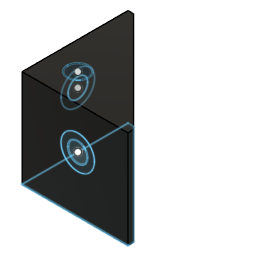
Electronics panel corner connector (Autodesk Fusion 360 design; units mm, degrees)
Autodesk Fusion 360 part; units mm, degrees
note: some values were not read from the file. Chosen so that the rebuilt part matches the saved one: which pieces of a blend or face edit are solid.
sketch "sketch 863" plane through (0, 28.398, 0) normal (0, -1, 0) x (-1, 0, 0)
  line L0 (-91, -772.5) -> (-73, -754.5)
  line L1 (-91, -773.5) -> (-91, -772.5)
  line L2 (-72, -773.5) -> (-91, -773.5)
  line L3 (-72, -773.5) -> (-91, -773.5)
  line L4 (-72, -754.5) -> (-72, -773.5)
  line L5 (-72, -754.5) -> (-72, -773.5)
  line L6 (-73, -754.5) -> (-72, -754.5)
extrude "Extrude1" add sketch "sketch 863" against normal blind 17.5
sketch "sketch 846" plane through (0, 45.898, 0) normal (0, 1, 0) x (-1, 0, 0)
  circle A0 centre (-77, 768.5) radius 1.875
extrude "Extrude2" cut sketch "sketch 846" against normal blind 7.5
sketch "sketch 893" plane through (0, 0, 773.5) normal (0, 0, 1) x (1, 0, 0)
  circle A0 centre (82, 38.398) radius 1.75
extrude "Extrude3" cut sketch "sketch 893" against normal blind 21
sketch "sketch 909" plane through (72, 0, 0) normal (-1, 0, 0) x (0, 0, 1)
  circle A0 centre (763.5, 38.398) radius 1.75
extrude "Extrude4" cut sketch "sketch 909" against normal blind 19
sketch "sketch 925" plane through (72, 0, 0) normal (-1, 0, 0) x (0, 0, 1)
  circle A0 centre (763.5, 38.398) radius 1.75
  circle A1 centre (763.5, 38.398) radius 3
extrude "Extrude5" cut sketch "sketch 925" against normal blind 8 from surface at -5
sketch "sketch 944" plane through (0, 0, 773.5) normal (0, 0, 1) x (1, 0, 0)
  circle A0 centre (82, 38.398) radius 1.75
  circle A1 centre (82, 38.398) radius 3
extrude "Extrude6" cut sketch "sketch 944" against normal blind 9 from surface at -5
chamfer "Chamfer2" distance 1.25 angle 45 2 edges at (80.3684, 39.0308, 768.5) (77, 39.0308, 761.8684)
chamfer "Chamfer3" distance 0.25 angle 45 2 edges at (85, 38.398, 766.5) (79, 38.398, 760.5)
